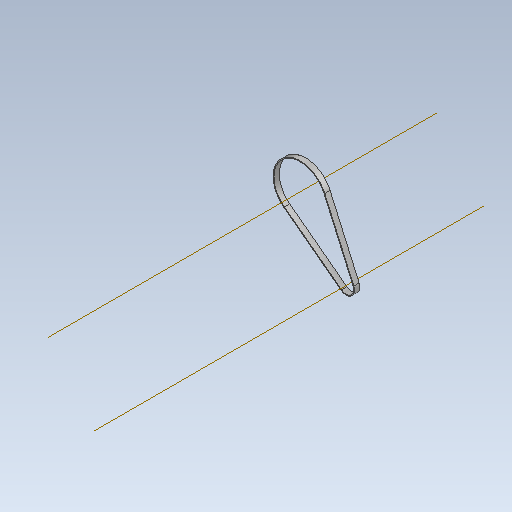
# Autodesk Inventor part: Synchronous Belt
Saved by Autodesk Inventor 2020 (Build 240168000, 168)
## iProperties
Created: 2021-05-22
Part Number: Synchronous Belt
Material: Rubber
Document SubType Name: Modeling
Designer: Iulian Bors
Density: 1 g/cm^3
Appearance: Rubber - Black - Version 1.1
CustomPartVersion: 1
Author: Iulian Bors
Autodesk Inventor part; units mm, degrees
sketch "Sketch Path" plane through (0, 0, 0) normal (0, 0, 1) x (1, 0, 0)
  arc A0 (-7.7036, 1.5124) -> (1.3498, 8.6927) centre (-4.1071, 6.2755) ccw
  arc A1 (-20.4174, 57.8328) -> (-50.5952, 33.8987) centre (-38.6071, 49.7755) ccw
  line L0 (-20.4174, 57.8328) -> (1.3498, 8.6927)
  line L1 (-7.7036, 1.5124) -> (-50.5952, 33.8987)
  constraints: 4 end point, 4 point on circle, 2 centre point
ref_plane "Cross Section Plane" through (1.3498, 8.6927, 0) normal (-0.405, 0.9143, 0) x (0, 0, 1)
ref_plane "Work Plane2" through (-4.1071, 6.2755, 0) normal (-1, 0, 0) x (0, 0, 1)
ref_plane "Work Plane3" through (-38.6071, 49.7755, 0) normal (0.7621, -0.6475, 0) x (0, 0, 1)
sketch "Cross Section" plane through (1.3498, 8.6927, 0) normal (-0.405, 0.9143, 0) x (0, 0, 1)
  line L0 (-2, 0.3) -> (2, 0.3)
  line L1 (2, 0.3) -> (2, -0.3)
  line L2 (2, -0.3) -> (-2, -0.3)
  line L3 (-2, -0.3) -> (-2, 0.3)
  line L4 (-2, 0) -> (2, 0) construction
  point P0 (0, 0)
  point P1 (0, 0)
  dimension "d0" = 4
  dimension "d4" = 0.3
  dimension "d5" = 0.3
  constraints: 10 end point, 3 midpoint, 2 parallel, 1 coincident, 1 horizontal, 1 perpendicular, 1 other
  measures "d0" distance between parallel lines of L1 L3
  measures "d4" distance between parallel lines of L2 L4
  measures "d5" distance between parallel lines of L4 L0
sweep "Belt" add profiles "Cross Section" path "Sketch Path"
equation "\"d0\" = da_B"
equation "\"d4\" = da_a"
equation "\"d5\" = da_a2"
equation "\"da_B\" = 4"
equation "\"da_pb\" = 2.5"
equation "\"da_L\" = 195.80225"
equation "\"da_a\" = 0.3"
equation "\"da_S\" = 1.5"
equation "\"da_Beta\" = 20deg"
equation "\"da_Ht\" = 0.7"
equation "\"da_H\" = 1.3"
equation "\"da_a2\" = 0.3"
body "Solid1"
